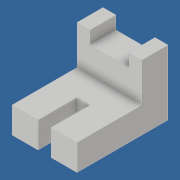
# Autodesk Inventor part: Part3
Saved by Autodesk Inventor 2018 (Build 220112000, 112)
## iProperties
Created: 2017-12-05
Part Number: Part3
Material: Generic
Document SubType Name: Modeling
Designer: 232963
Density: 1 g/cm^3
Appearance: Default
Author: 232963
Autodesk Inventor part; units mm, degrees
ref_plane "YZ Plane" through (0, 0, 0) normal (1, 0, 0) x (0, 1, 0)
ref_plane "XZ Plane" through (0, 0, 0) normal (0, 1, 0) x (-1, 0, 0)
ref_plane "XY Plane" through (0, 0, 0) normal (0, 0, 1) x (1, 0, 0)
sketch "Sketch1" plane through (0, 0, 0) normal (0, 1, 0) x (-1, 0, 0)
  line L0 (30.1994, -90.5323) -> (-33.3006, -90.5323)
  line L1 (-33.3006, -90.5323) -> (-33.3006, -1.6323)
  line L2 (30.1994, -1.6323) -> (30.1994, -90.5323)
  line L3 (-7.9006, -1.6323) -> (-7.9006, -39.7323)
  line L4 (-7.9006, -39.7323) -> (4.7994, -39.7323)
  line L5 (4.7994, -39.7323) -> (4.7994, -1.6323)
  line L6 (-33.3006, -1.6323) -> (-7.9006, -1.6323)
  line L7 (4.7994, -1.6323) -> (30.1994, -1.6323)
  point P0 (0, 0)
  dimension "d0" = 63.5
  dimension "d1" = 88.9
  dimension "d2" = 25.4
  dimension "d3" = 25.4
  dimension "d4" = 38.1
  constraints: 16 end point, 4 parallel, 1 horizontal, 1 perpendicular
  measures "d0" distance of L1.end L2.start
  measures "d1" distance of L0.end L1.end
  measures "d2" distance of L5.end L2.start
  measures "d3" distance of L1.end L3.start
  measures "d4" distance of L4.end L5.end
extrude "Extrusion1" add sketch "Sketch1" along normal blind 25.4
sketch "Sketch2" plane through (0, 25.4, 0) normal (0, 1, 0) x (1, 0, 0)
  line L0 (-30.1994, 90.5323) -> (-30.1994, 1.6323) projected
  line L1 (33.3006, 1.6323) -> (33.3006, 90.5323) projected
  line L2 (-30.1994, 90.5323) -> (33.3006, 90.5323)
  line L3 (33.3006, 90.5323) -> (33.3006, 65.1323)
  line L4 (33.3006, 65.1323) -> (-30.1994, 65.1323)
  line L5 (-30.1994, 65.1323) -> (-30.1994, 90.5323)
  point P0 (0, 0)
  dimension "d7" = 25.4
  constraints: 8 end point, 2 parallel, 1 horizontal, 1 perpendicular, 1 point on line
  measures "d7" distance between parallel lines of L2 L4
extrude "Extrusion2" add sketch "Sketch2" along normal blind 38.1
sketch "Sketch3" plane through (0, 63.5, 0) normal (0, 1, 0) x (1, 0, 0)
  line L0 (-30.1994, 90.5323) -> (33.3006, 90.5323) projected
  line L1 (-17.4994, 90.5323) -> (20.6006, 90.5323)
  line L2 (20.6006, 90.5323) -> (20.6006, 65.1323)
  line L3 (20.6006, 65.1323) -> (-17.4994, 65.1323)
  line L4 (-17.4994, 65.1323) -> (-17.4994, 90.5323)
  line L5 (-30.1994, 90.5323) -> (-30.1994, 65.1323) projected
  point P0 (0, 0)
  dimension "d10" = 25.4
  dimension "d11" = 12.7
  dimension "d13" = 38.1
  constraints: 8 end point, 2 parallel, 1 horizontal, 1 perpendicular, 1 point on line
  measures "d10" distance of L3.end L1.start
  measures "d11" distance between parallel lines of L5 L4
  measures "d13" distance between parallel lines of L2 L4
extrude "Extrusion3" cut sketch "Sketch3" against normal blind 12.7
body "Solid1"
